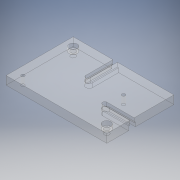
# Autodesk Inventor part: PCB FIxture 80x40
Saved by Autodesk Inventor 2017 (Build 210142000, 142)
## iProperties
Created: 2016-09-16
Part Number: PCB FIxture 80x40
Material: Polycarbonate, Clear
Document SubType Name: Modeling
Designer: Andreas Fröderberg
Density: 1.2 g/cm^3
Appearance: Polycarbonate - Clear
Author: Andreas Fröderberg
Autodesk Inventor part; units mm, degrees
ref_plane "YZ Plane" through (0, 0, 0) normal (1, 0, 0) x (0, 1, 0)
ref_plane "XZ Plane" through (0, 0, 0) normal (0, 1, 0) x (-1, 0, 0)
ref_plane "XY Plane" through (0, 0, 0) normal (0, 0, 1) x (1, 0, 0)
sketch "Sketch1" plane through (0, 0, 0) normal (0, 0, 1) x (1, 0, 0)
  line L0 (-10, -10) -> (110, -10)
  line L1 (110, -10) -> (110, 70)
  line L2 (110, 70) -> (-10, 70)
  line L3 (-10, 70) -> (-10, -10)
  point P0 (0, 0)
  dimension "W_tot" = 120
  dimension "H_tot" = 80
  dimension "E_to_Hole_X" = 10
  dimension "E_to_Hole_Y" = 10
  constraints: 8 end point, 2 parallel, 1 horizontal, 1 perpendicular
  measures "W_tot" distance of L1.end L2.end
  measures "H_tot" distance of L2.end L0.start
  measures "E_to_Hole_X" distance from line of L3 point (0, 0)
  measures "E_to_Hole_Y" distance from line of L0 point (0, 0)
extrude "Body_Ex" add sketch "Sketch1" against normal blind 10
sketch "Hole_4_sk" plane through (0, 0, 0) normal (0, 0, 1) x (1, 0, 0)
  line L0 (0, 0) -> (80, 0) construction
  line L1 (80, 0) -> (80, 40) construction
  line L2 (80, 40) -> (0, 40) construction
  line L3 (0, 40) -> (0, 0) construction
  point P0 (80, 40)
  dimension "CP_Hole_X" = 80
  dimension "CP_Hole_Y" = 40
  constraints: 8 end point, 2 coincident, 2 parallel, 1 horizontal, 1 perpendicular
  measures "CP_Hole_X" distance of L1.end L2.end
  measures "CP_Hole_Y" distance of L0.end L1.end
hole "Hole1" at (80, 40, 0) at (0, 0, 0) direction (0, 0, -1) diameter 4 end through all
sketch "Lock Track Profile" plane through (110, -10, 0) normal (1, 0, 0) x (0, 0, -1)
  line L0 (0, 27.4) -> (5, 27.4)
  line L1 (5, 27.4) -> (5, 25.9)
  line L2 (5, 25.9) -> (10, 25.9)
  line L3 (10, 25.9) -> (10, 34.1)
  line L4 (10, 34.1) -> (5, 34.1)
  line L5 (5, 34.1) -> (5, 32.6)
  line L6 (5, 32.6) -> (0, 32.6)
  line L7 (0, 32.6) -> (0, 27.4)
  line L8 (0, 0) -> (0, 80) projected
  line L9 (10, 80) -> (10, 0) projected
  point P0 (0, 10)
  dimension "Lock_Track_W" = 5.2
  dimension "Lock_Track_Bolt_W" = 8.2
  dimension "Origin_to_lock_track" = 15.9
  constraints: 16 end point, 6 perpendicular, 2 collinear, 2 equal length, 2 horizontal, 1 vertical alignment
  measures "Lock_Track_W" distance of L6.end L0.start
  measures "Lock_Track_Bolt_W" distance of L2.end L3.end
  measures "Origin_to_lock_track" distance from line of L2 point (0, 10)
sketch "Sketch5" plane through (0, 0, 0) normal (0, 0, 1) x (1, 0, 0)
  line L0 (75, 20) -> (110, 20)
  line L1 (110, -10) -> (110, 70) projected
  circle A0 centre (80, 40) radius 2 projected
  point P0 (0, 0)
  dimension "d19" = 20
  dimension "d20" = 5
  constraints: 2 end point, 1 horizontal, 1 point on line
  measures "d19" distance from line of L0 point (0, 0)
  measures "d20" horizontal distance of L0.start A0.centre
sweep "Lock track" cut profiles "Lock Track Profile" path "Sketch5" path curves L0
full round fillet "Lock track fillet small" first side at (98.3333, 22.6, -3.3333) centre faces at (75, 20.8667, -8.3333) second side at (98.3333, 17.4, -1.6667)
full round fillet "Lock track fillet large" first side at (98.3333, 24.1, -8.3333) centre faces at (75, 20, -8.3333) second side at (98.3333, 15.9, -6.6667)
sketch "Lock track Y" plane through (-10, 70, 0) normal (0, 1, 0) x (1, 0, 0)
  line L0 (52.6, 0) -> (47.4, 0)
  line L1 (47.4, 0) -> (47.4, 5)
  line L2 (47.4, 5) -> (45.9, 5)
  line L3 (45.9, 5) -> (45.9, 10)
  line L4 (45.9, 10) -> (54.1, 10)
  line L5 (54.1, 10) -> (54.1, 5)
  line L6 (54.1, 5) -> (52.6, 5)
  line L7 (52.6, 5) -> (52.6, 0)
  line L8 (0, 10) -> (120, 10) projected
  line L9 (120, 0) -> (0, 0) projected
  point P0 (10, 0)
  dimension "d23" = 8.2
  dimension "d24" = 5.2
  dimension "d25" = 5
  dimension "d26" = 35.9
  constraints: 16 end point, 6 perpendicular, 3 collinear, 2 point on line, 1 horizontal, 1 horizontal alignment
  measures "d23" distance of L3.end L4.end
  measures "d24" distance of L0.start L0.end
  measures "d25" distance of L4.end L5.end
  measures "d26" distance from line of L3 point (10, 0)
sketch "Lock track 2 Profile" plane through (0, 0, 0) normal (0, 0, 1) x (1, 0, 0)
  line L0 (40, 70) -> (40, 35)
  line L1 (110, 70) -> (-10, 70) projected
  circle A0 centre (80, 40) radius 2 projected
  point P0 (0, 0)
  dimension "d27" = 5
  dimension "d28" = 40
  constraints: 2 end point, 1 point on line, 1 vertical
  measures "d27" vertical distance of L0.end A0.centre
  measures "d28" distance from line of point (0, 0) L0
sweep "Sweep2" cut profiles "Lock track Y" path "Lock track 2 Profile" path curves L0
full round fillet "Fillet3" first side at (42.6, 46.6667, -1.6667) centre faces at (40.8667, 35, -8.3333) second side at (37.4, 46.6667, -3.3333)
full round fillet "Fillet4" first side at (44.1, 46.6667, -6.6667) centre faces at (40, 35, -8.3333) second side at (35.9, 46.6667, -8.3333)
sketch "Sketch9" plane through (0, 0, 0) normal (0, 0, 1) x (1, 0, 0)
  line L0 (-10, 70) -> (-10, -10) projected
  line L1 (-10, 70) -> (35.9, 70) projected
  line L2 (-10, -10) -> (110, -10) projected
  line L3 (110, -10) -> (110, 17.4) projected
  point P0 (0, 0)
  point P1 (0, 60)
  point P2 (100, 0)
  dimension "d31" = 10
  dimension "d32" = 10
  dimension "d33" = 10
  dimension "d34" = 10
  measures "d31" distance from line of L0 point (0, 60)
  measures "d32" distance from line of L1 point (0, 60)
  measures "d33" distance from line of point (100, 0) L2
  measures "d34" distance from line of point (100, 0) L3
hole "Hole2" at (0, 60, 0) at (100, 0, 0) direction (0, 0, -1) diameter 5.7 end through all counterbore diameter 9.75 counterbore depth 5
equation "\"Origin_to_lock_track\" = 0.5 * CP_Hole_Y - 0.5 * Lock_Track_Bolt_W"
equation "\"d19\" = 0.5 * CP_Hole_Y"
equation "\"d23\" = Lock_Track_Bolt_W"
equation "\"d24\" = Lock_Track_W"
equation "\"d25\" = 0.5 * T_Base_Ex"
equation "\"d26\" = 0.5 * CP_Hole_X - 0.5 * Lock_Track_Bolt_W"
equation "\"d28\" = 0.5 * CP_Hole_X"
equation "\"T_Base_Ex\" = 10"
